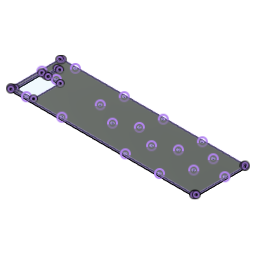
bot_plate_2 (Autodesk Fusion 360 design; units mm, degrees)
Autodesk Fusion 360 part; units mm, degrees
sketch "Sketch1" plane through (0, 0, 0) normal (0, 0, 1) x (1, 0, 0)
  circle A0 centre (317.6723, -113.9909) radius 1.5
  circle A1 centre (386.7293, -18.6469) radius 1.5
  line L0 (30.0243, -116.3719) -> (386.7293, -116.3719)
  circle A2 centre (229.5683, -18.5529) radius 1.5
  circle A3 centre (262.9063, -74.7719) radius 1.5
  line L1 (389.2043, -113.8969) -> (389.2043, -18.6469)
  arc A4 (389.2043, -18.6469) -> (386.7293, -16.1719) centre (386.7293, -18.6469) ccw
  circle A5 centre (143.8433, -55.7219) radius 1.5
  circle A6 centre (296.2433, -55.7219) radius 1.5
  line L2 (386.7293, -16.1719) -> (30.0243, -16.1719)
  circle A7 centre (305.7683, -18.5529) radius 1.5
  circle A8 centre (386.7293, -55.7219) radius 1.5
  circle A9 centre (153.3663, -18.5529) radius 1.5
  arc A10 (27.6433, -113.9909) -> (30.0243, -116.3719) centre (30.0243, -113.9909) ccw
  circle A11 centre (58.0243, -55.7219) radius 1.5
  circle A12 centre (30.0243, -18.5529) radius 1.5
  circle A13 centre (250.9983, -113.9909) radius 1.5
  line L3 (27.6433, -18.5529) -> (27.6433, -113.9909)
  circle A14 centre (58.0243, -18.5529) radius 1.5
  arc A15 (30.0243, -16.1719) -> (27.6433, -18.5529) centre (30.0243, -18.5529) ccw
  circle A16 centre (127.1733, -113.9909) radius 1.5
  arc A17 (386.7293, -116.3719) -> (389.2043, -113.8969) centre (386.7293, -113.8969) ccw
  circle A18 centre (386.7293, -113.8969) radius 1.5
  circle A19 centre (30.0243, -55.7219) radius 1.5
  circle A20 centre (345.1433, -74.7719) radius 1.5
  circle A21 centre (30.0243, -113.9909) radius 1.5
  circle A22 centre (220.0433, -55.7219) radius 1.5
  circle A23 centre (58.0243, -113.9909) radius 1.5
  circle A24 centre (186.7063, -74.7719) radius 1.5
  circle A25 centre (345.1433, -36.6719) radius 1.5
  point P0 (389.2043, -16.1719)
  point P1 (27.6433, -16.1719)
  point P2 (389.2043, -116.3719)
  dimension "d78" = 100.2
  dimension "d79" = 361.561
  dimension "d80" = 3
  dimension "d81" = 2.381
  dimension "d82" = 2.381
  dimension "d83" = 30.381
  dimension "d84" = 125.723
  dimension "d85" = 201.925
  dimension "d86" = 278.125
  dimension "d87" = 2.475
  dimension "d88" = 2.475
  dimension "d89" = 2.381
  dimension "d90" = 2.381
  dimension "d91" = 2.381
  dimension "d92" = 2.381
  dimension "d93" = 3
  dimension "d94" = 3
  dimension "d95" = 3
  dimension "d96" = 3
  dimension "d97" = 3
  dimension "d98" = 2.381
  dimension "d99" = 2.381
  dimension "d100" = 2.381
  dimension "d101" = 2.381
  dimension "d102" = 2.381
  dimension "d103" = 2.381
  dimension "d104" = 2.381
  dimension "d105" = 2.475
  dimension "d106" = 2.475
  dimension "d107" = 2.475
  dimension "d108" = 39.55
  dimension "d109" = 39.55
  dimension "d110" = 39.55
  dimension "d111" = 39.55
  dimension "d112" = 39.55
  dimension "d113" = 39.55
  dimension "d114" = 30.381
  dimension "d115" = 116.2
  dimension "d116" = 192.4
  dimension "d117" = 268.6
  dimension "d118" = 44.061
  dimension "d119" = 20.5
  dimension "d120" = 3
  dimension "d121" = 3
  dimension "d122" = 3
  dimension "d123" = 3
  dimension "d124" = 3
  dimension "d125" = 3
  dimension "d126" = 30.381
  dimension "d127" = 99.53
  dimension "d128" = 223.355
  dimension "d129" = 290.029
  dimension "d130" = 44.061
  dimension "d131" = 58.6
  dimension "d132" = 159.063
  dimension "d133" = 235.263
  dimension "d134" = 41.6
  dimension "d135" = 41.6
  dimension "d136" = 3
  dimension "d137" = 3
  dimension "d138" = 3
  dimension "d139" = 3
  dimension "d140" = 3
  dimension "d141" = 3
  dimension "d142" = 3
  dimension "d143" = 3
  dimension "d144" = 3
  dimension "d145" = 3
  dimension "d146" = 2.381
  dimension "d147" = 2.381
  dimension "d148" = 2.475
  dimension "d149" = 2.475
  constraint horizontal L2
  constraint vertical L3
  constraint horizontal L0
  constraint vertical L1
  constraint coincident P1 L2
  constraint coincident P1 L3
  constraint tangent L2 A15
  constraint tangent L3 A15
  constraint tangent A10 L3
  constraint tangent L0 A10
  constraint coincident P2 L1
  constraint coincident P2 L0
  constraint tangent L1 A17
  constraint tangent L0 A17
  constraint coincident P0 L1
  constraint coincident P0 L2
  constraint tangent L1 A4
  constraint tangent A4 L2
  measures "d78" distance of P0 P2
  measures "d79" distance of P0 P1
  measures "d80" diameter of A12
  measures "d81" distance of A12.centre L2
  measures "d82" distance of A12.centre L3
  measures "d83" distance of A14.centre L3
  measures "d84" distance of A9.centre L3
  measures "d85" distance of A2.centre L3
  measures "d86" distance of A7.centre L3
  measures "d87" distance of A1.centre L2
  measures "d88" distance of A1.centre L1
  measures "d89" distance of A7.centre L2
  measures "d90" distance of A2.centre L2
  measures "d91" distance of A9.centre L2
  measures "d92" distance of A14.centre L2
  measures "d93" diameter of A14
  measures "d94" diameter of A9
  measures "d95" diameter of A2
  measures "d96" diameter of A7
  measures "d97" diameter of A1
  measures "d98" distance of A19.centre L3
  measures "d99" distance of A10.centre L3
  measures "d100" distance of A10.centre L0
  measures "d101" distance of A23.centre L0
  measures "d102" distance of A16.centre L0
  measures "d103" distance of A13.centre L0
  measures "d104" distance of A0.centre L0
  measures "d105" distance of A17.centre L0
  measures "d106" distance of A17.centre L1
  measures "d107" distance of A8.centre L1
  measures "d108" distance of A19.centre L2
  measures "d109" distance of A11.centre L2
  measures "d110" distance of A5.centre L2
  measures "d111" distance of A22.centre L2
  measures "d112" distance of A6.centre L2
  measures "d113" distance of A8.centre L2
  measures "d114" distance of A11.centre L3
  measures "d115" distance of A5.centre L3
  measures "d116" distance of A22.centre L3
  measures "d117" distance of A6.centre L3
  measures "d118" distance of A25.centre L1
  measures "d119" distance of A25.centre L2
  measures "d120" diameter of A25
  measures "d121" diameter of A6
  measures "d122" diameter of A22
  measures "d123" diameter of A5
  measures "d124" diameter of A11
  measures "d125" diameter of A19
  measures "d126" distance of A23.centre L3
  measures "d127" distance of A16.centre L3
  measures "d128" distance of A13.centre L3
  measures "d129" distance of A0.centre L3
  measures "d130" distance of A20.centre L1
  measures "d131" distance of A20.centre L2
  measures "d132" distance of A24.centre L3
  measures "d133" distance of A3.centre L3
  measures "d134" distance of A24.centre L0
  measures "d135" distance of A3.centre L0
  measures "d136" diameter of A24
  measures "d137" diameter of A20
  measures "d138" diameter of A8
  measures "d139" diameter of A18
  measures "d140" diameter of A0
  measures "d141" diameter of A3
  measures "d142" diameter of A13
  measures "d143" diameter of A16
  measures "d144" diameter of A23
  measures "d145" diameter of A21
  measures "d146" radius of A15
  measures "d147" radius of A10
  measures "d148" radius of A17
  measures "d149" radius of A4
extrude "Extrude1" add sketch "Sketch1" along normal blind 3
sketch "Sketch2" plane through (0, 0, 3) normal (0, 0, 1) x (-1, 0, 0)
  circle A0 centre (-143.8433, 55.7219) radius 1.5
  circle A1 centre (-386.7293, 113.8969) radius 1.5
  circle A2 centre (-262.9063, 74.7719) radius 1.5
  circle A3 centre (-30.0243, 113.9909) radius 1.5
  circle A4 centre (-58.0243, 55.7219) radius 1.5
  circle A5 centre (-250.9983, 113.9909) radius 1.5
  circle A6 centre (-317.6723, 113.9909) radius 1.5
  circle A7 centre (-296.2433, 55.7219) radius 1.5
  circle A8 centre (-127.1733, 113.9909) radius 1.5
  circle A9 centre (-386.7293, 55.7219) radius 1.5
  circle A10 centre (-386.7293, 18.6469) radius 1.5
  circle A11 centre (-345.1433, 74.7719) radius 1.5
  circle A12 centre (-58.0243, 18.5529) radius 1.5
  circle A13 centre (-30.0243, 18.5529) radius 1.5
  circle A14 centre (-186.7063, 74.7719) radius 1.5
  circle A15 centre (-345.1433, 36.6719) radius 1.5
  circle A16 centre (-153.3663, 18.5529) radius 1.5
  circle A17 centre (-305.7683, 18.5529) radius 1.5
  circle A18 centre (-229.5683, 18.5529) radius 1.5
  circle A19 centre (-58.0243, 113.9909) radius 1.5
  circle A20 centre (-30.0243, 55.7219) radius 1.5
  circle A21 centre (-220.0433, 55.7219) radius 1.5
  arc A22 (-386.7293, 116.3719) -> (-389.2043, 113.8969) centre (-386.7293, 113.8969) ccw
  line L0 (-389.2043, 113.8969) -> (-389.2043, 18.6469)
  arc A23 (-389.2043, 18.6469) -> (-386.7293, 16.1719) centre (-386.7293, 18.6469) ccw
  line L1 (-386.7293, 16.1719) -> (-30.0243, 16.1719)
  arc A24 (-30.0243, 16.1719) -> (-27.6433, 18.5529) centre (-30.0243, 18.5529) ccw
  line L2 (-27.6433, 18.5529) -> (-27.6433, 113.9909)
  arc A25 (-27.6433, 113.9909) -> (-30.0243, 116.3719) centre (-30.0243, 113.9909) ccw
  line L3 (-30.0243, 116.3719) -> (-386.7293, 116.3719)
  line L4 (-32.6433, 58.7219) -> (-68.6433, 58.7219)
  line L5 (-68.6433, 58.7219) -> (-68.6433, 110.7219)
  line L6 (-68.6433, 110.7219) -> (-32.6433, 110.7219)
  line L7 (-32.6433, 110.7219) -> (-32.6433, 58.7219)
  line L8 (-40, 36.1719) -> (-45, 36.1719)
  line L9 (-45, 36.1719) -> (-45, 58.7219)
  line L10 (-45, 58.7219) -> (-40, 58.7219)
  line L11 (-40, 58.7219) -> (-40, 36.1719)
  dimension "d153" = 36
  dimension "d154" = 52
  dimension "d155" = 3
  dimension "d156" = 5
  dimension "d159" = 5
  dimension "d161" = 20
  constraint horizontal L4
  constraint vertical L5
  constraint horizontal L6
  constraint vertical L7
  constraint horizontal L8
  constraint vertical L9
  constraint horizontal L10
  constraint vertical L11
  constraint coincident L4 L9.end
  measures "d153" distance of L4.start L4.end
  measures "d154" distance of L4.start L6.end
  measures "d155" distance of A4.centre L4
  measures "d156" distance of L2 L7
  measures "d159" distance of L8.start L8.end
  measures "d161" distance of L1 L8
extrude "Extrude2" cut sketch "Sketch2" against normal blind 3 contours L4 L5 L6 L7 L10 | L4 L8 L9 L10 L11
sketch "Sketch3" plane through (0, 0, 3) normal (0, 0, 1) x (-1, 0, 0)
  line L0 (-68.6433, 58.7219) -> (-68.6433, 110.7219)
  line L1 (-68.6433, 110.7219) -> (-32.6433, 110.7219)
  line L2 (-32.6433, 110.7219) -> (-32.6433, 58.7219)
  line L3 (-32.6433, 58.7219) -> (-40, 58.7219)
  circle A0 centre (-143.8433, 55.7219) radius 1.5
  circle A1 centre (-386.7293, 113.8969) radius 1.5
  circle A2 centre (-262.9063, 74.7719) radius 1.5
  circle A3 centre (-30.0243, 113.9909) radius 1.5
  circle A4 centre (-58.0243, 55.7219) radius 1.5
  circle A5 centre (-250.9983, 113.9909) radius 1.5
  circle A6 centre (-317.6723, 113.9909) radius 1.5
  circle A7 centre (-296.2433, 55.7219) radius 1.5
  circle A8 centre (-127.1733, 113.9909) radius 1.5
  circle A9 centre (-386.7293, 55.7219) radius 1.5
  circle A10 centre (-386.7293, 18.6469) radius 1.5
  circle A11 centre (-345.1433, 74.7719) radius 1.5
  circle A12 centre (-58.0243, 18.5529) radius 1.5
  circle A13 centre (-30.0243, 18.5529) radius 1.5
  circle A14 centre (-186.7063, 74.7719) radius 1.5
  circle A15 centre (-345.1433, 36.6719) radius 1.5
  circle A16 centre (-153.3663, 18.5529) radius 1.5
  circle A17 centre (-305.7683, 18.5529) radius 1.5
  circle A18 centre (-229.5683, 18.5529) radius 1.5
  circle A19 centre (-58.0243, 113.9909) radius 1.5
  circle A20 centre (-30.0243, 55.7219) radius 1.5
  circle A21 centre (-220.0433, 55.7219) radius 1.5
  arc A22 (-386.7293, 116.3719) -> (-389.2043, 113.8969) centre (-386.7293, 113.8969) ccw
  line L4 (-389.2043, 113.8969) -> (-389.2043, 18.6469)
  arc A23 (-389.2043, 18.6469) -> (-386.7293, 16.1719) centre (-386.7293, 18.6469) ccw
  line L5 (-386.7293, 16.1719) -> (-30.0243, 16.1719)
  arc A24 (-30.0243, 16.1719) -> (-27.6433, 18.5529) centre (-30.0243, 18.5529) ccw
  line L6 (-27.6433, 18.5529) -> (-27.6433, 113.9909)
  arc A25 (-27.6433, 113.9909) -> (-30.0243, 116.3719) centre (-30.0243, 113.9909) ccw
  line L7 (-30.0243, 116.3719) -> (-386.7293, 116.3719)
  line L8 (-40, 58.7219) -> (-40, 36.1719)
  line L9 (-40, 36.1719) -> (-45, 36.1719)
  line L10 (-45, 36.1719) -> (-45, 58.7219)
  line L11 (-45, 58.7219) -> (-68.6433, 58.7219)
sketch "Sketch4" plane through (0, 0, 3) normal (0, 0, 1) x (-1, 0, 0)
  line L0 (-68.6433, 58.7219) -> (-68.6433, 110.7219)
  line L1 (-68.6433, 110.7219) -> (-32.6433, 110.7219)
  line L2 (-32.6433, 110.7219) -> (-32.6433, 58.7219)
  line L3 (-32.6433, 58.7219) -> (-40, 58.7219)
  circle A0 centre (-143.8433, 55.7219) radius 1.5
  circle A1 centre (-386.7293, 113.8969) radius 1.5
  circle A2 centre (-262.9063, 74.7719) radius 1.5
  circle A3 centre (-30.0243, 113.9909) radius 1.5
  circle A4 centre (-58.0243, 55.7219) radius 1.5
  circle A5 centre (-250.9983, 113.9909) radius 1.5
  circle A6 centre (-317.6723, 113.9909) radius 1.5
  circle A7 centre (-296.2433, 55.7219) radius 1.5
  circle A8 centre (-127.1733, 113.9909) radius 1.5
  circle A9 centre (-386.7293, 55.7219) radius 1.5
  circle A10 centre (-386.7293, 18.6469) radius 1.5
  circle A11 centre (-345.1433, 74.7719) radius 1.5
  circle A12 centre (-58.0243, 18.5529) radius 1.5
  circle A13 centre (-30.0243, 18.5529) radius 1.5
  circle A14 centre (-186.7063, 74.7719) radius 1.5
  circle A15 centre (-345.1433, 36.6719) radius 1.5
  circle A16 centre (-153.3663, 18.5529) radius 1.5
  circle A17 centre (-305.7683, 18.5529) radius 1.5
  circle A18 centre (-229.5683, 18.5529) radius 1.5
  circle A19 centre (-58.0243, 113.9909) radius 1.5
  circle A20 centre (-30.0243, 55.7219) radius 1.5
  circle A21 centre (-220.0433, 55.7219) radius 1.5
  arc A22 (-386.7293, 116.3719) -> (-389.2043, 113.8969) centre (-386.7293, 113.8969) ccw
  line L4 (-389.2043, 113.8969) -> (-389.2043, 18.6469)
  arc A23 (-389.2043, 18.6469) -> (-386.7293, 16.1719) centre (-386.7293, 18.6469) ccw
  line L5 (-386.7293, 16.1719) -> (-30.0243, 16.1719)
  arc A24 (-30.0243, 16.1719) -> (-27.6433, 18.5529) centre (-30.0243, 18.5529) ccw
  line L6 (-27.6433, 18.5529) -> (-27.6433, 113.9909)
  arc A25 (-27.6433, 113.9909) -> (-30.0243, 116.3719) centre (-30.0243, 113.9909) ccw
  line L7 (-30.0243, 116.3719) -> (-386.7293, 116.3719)
  line L8 (-40, 58.7219) -> (-40, 36.1719)
  line L9 (-40, 36.1719) -> (-45, 36.1719)
  line L10 (-45, 36.1719) -> (-45, 58.7219)
  line L11 (-45, 58.7219) -> (-68.6433, 58.7219)
equation "d80 = m2_hole_standoff"
equation "d93 = m2_hole_standoff"
equation "d94 = m2_hole_standoff"
equation "d95 = m2_hole_standoff"
equation "d96 = m2_hole_standoff"
equation "d97 = m2_hole_standoff"
equation "d120 = m2_hole_standoff"
equation "d121 = m2_hole_standoff"
equation "d122 = m2_hole_standoff"
equation "d123 = m2_hole_standoff"
equation "d124 = m2_hole_standoff"
equation "d125 = m2_hole_standoff"
equation "d136 = m2_hole_standoff"
equation "d137 = m2_hole_standoff"
equation "d138 = m2_hole_standoff"
equation "d139 = m2_hole_standoff"
equation "d140 = m2_hole_standoff"
equation "d141 = m2_hole_standoff"
equation "d142 = m2_hole_standoff"
equation "d143 = m2_hole_standoff"
equation "d144 = m2_hole_standoff"
equation "d145 = m2_hole_standoff"
equation "m2_hole_standoff = 3 mm"
